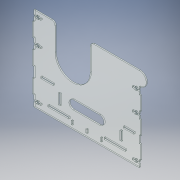
# Autodesk Inventor part: Lat_Izq_Caja
Saved by Autodesk Inventor 2019 (Build 230136000, 136)
## iProperties
Created: 2020-04-06
Part Number: Lat_Izq_Caja
Material: Generic
Document SubType Name: Modeling
Designer: Jurgen
Density: 1 g/cm^3
Appearance: Clear
Author: Jurgen
Autodesk Inventor part; units mm, degrees
ref_plane "YZ Plane" through (0, 0, 0) normal (1, 0, 0) x (0, 1, 0)
ref_plane "XZ Plane" through (0, 0, 0) normal (0, 1, 0) x (-1, 0, 0)
ref_plane "XY Plane" through (0, 0, 0) normal (0, 0, 1) x (1, 0, 0)
sketch "Sketch1" plane through (0, 0, 0) normal (0, 0, 1) x (1, 0, 0)
  line L0 (-150, -102.5) -> (40, -102.5) construction
  line L1 (-150, 5) -> (-150, -102.5) construction
  line L2 (-130, -37.5) -> (-95, -37.5)
  line L3 (-95, -37.5) -> (-95, -42.5)
  line L4 (-95, -42.5) -> (-130, -42.5)
  line L5 (-130, -37.5) -> (-130, -42.5)
  line L6 (-110, -97.5) -> (-50, -97.5)
  line L7 (-110, -97.5) -> (-110, -102.5)
  line L8 (-50, -102.5) -> (-110, -102.5)
  line L9 (-50, -97.5) -> (-50, -102.5)
  line L10 (110, -97.5) -> (50, -97.5)
  line L11 (110, -102.5) -> (50, -102.5)
  line L12 (50, -97.5) -> (50, -102.5)
  line L13 (110, -97.5) -> (110, -102.5)
  line L14 (95, -82.5) -> (95, -57.5)
  line L15 (95, -57.5) -> (100, -57.5)
  line L16 (100, -57.5) -> (100, -82.5)
  line L17 (95, -82.5) -> (100, -82.5)
  line L18 (-80, -82.5) -> (-80, -52.5)
  line L19 (-75, -52.5) -> (-75, -82.5)
  line L20 (-80, -52.5) -> (-75, -52.5)
  line L21 (-80, -82.5) -> (-75, -82.5)
  line L22 (135, -47.5) -> (105, -47.5)
  line L23 (135, -42.5) -> (105, -42.5)
  line L24 (105, -42.5) -> (105, -47.5)
  line L25 (135, -42.5) -> (135, -47.5)
  line L26 (-150, -97.5) -> (-150, -102.5) construction
  line L27 (-110, -102.5) -> (-150, -102.5) construction
  line L28 (150, -102.5) -> (110, -102.5) construction
  line L29 (150, -97.5) -> (150, -102.5) construction
  circle A0 centre (-39.5, 42.5) radius 33.5 construction
  circle A1 centre (-39.5, 42.5) radius 21 construction
  arc A2 (-27.2498, 9) -> (-19.0518, 13.2735) centre (-27.2498, 19) ccw construction
  line L30 (-27.2498, 9) -> (-81.7502, 9) construction
  line L31 (-1.6215, 38.2265) -> (-19.0518, 13.2735) construction
  arc A3 (6.5765, 42.5) -> (-1.6215, 38.2265) centre (6.5765, 32.5) ccw construction
  arc A4 (-89.9482, 13.2735) -> (-81.7502, 9) centre (-81.7502, 19) ccw construction
  line L32 (-89.9482, 13.2735) -> (-107.3785, 38.2265) construction
  arc A5 (-107.3785, 38.2265) -> (-115.5765, 42.5) centre (-115.5765, 32.5) ccw construction
  line L33 (-150, -102.5) -> (150, -102.5) construction
  line L34 (150, -102.5) -> (150, 117.5) construction
  line L35 (150, 117.5) -> (-150, 117.5) construction
  line L36 (-150, 117.5) -> (-150, -102.5) construction
  line L37 (-150, -102.5) -> (150, -102.5) construction
  line L38 (150, -102.5) -> (150, -122.5) construction
  line L39 (150, -122.5) -> (-150, -122.5)
  line L40 (-150, -122.5) -> (-150, -102.5) construction
  line L41 (-150, -122.5) -> (-150, 117.5)
  line L42 (150, 117.5) -> (150, -122.5)
  circle A6 centre (-39.5, 42.5) radius 50 construction
  line L43 (-150, 117.5) -> (-115.5765, 117.5) construction
  line L44 (-150, 117.5) -> (-120, 117.5)
  line L45 (46.1387, 117.5) -> (150, 117.5)
  line L46 (-89.5, 42.5) -> (10.5, 42.5) construction
  line L47 (-89.5, 42.5) -> (-89.5, 117.5) construction
  line L48 (10.5, 42.5) -> (10.5, 117.5) construction
  line L49 (-120, 117.5) -> (-89.5, 117.5)
  line L50 (-89.5, 117.5) -> (-89.5, 42.5)
  line L51 (46.1387, 117.5) -> (10.5, 117.5)
  line L52 (10.5, 117.5) -> (10.5, 42.5)
  arc A7 (-89.5, 42.5) -> (10.5, 42.5) centre (-39.5, 42.5) ccw
  point P0 (0, 0)
  point P1 (-84.8873, 21.524)
  point P2 (4.6333, 19)
  dimension "d2" = 300
  dimension "d3" = 220
  dimension "d4" = 300
  dimension "d5" = 20
  dimension "d6" = 100
  dimension "d7" = 30
  constraints: 106 end point, 14 point on circle, 8 centre point, 5 horizontal, 5 perpendicular, 5 point on line, 4 parallel, 2 collinear, 2 tangent, 1 coincident
  measures "d2" distance of L35.end L34.end
  measures "d3" distance of L34.end L33.end
  measures "d4" distance of L38.end L39.end
  measures "d5" distance of L37.end L38.end
  measures "d6" diameter of A6
  measures "d7" distance of L35.end L44.end
extrude "Extrusion1" add sketch "Sketch1" along normal blind 3.5
fillet "Fillet1" radius 10 2 edges at (-89.5, 117.5, 1.75) (10.5, 117.5, 1.75)
sketch "Sketch4" plane through (0, 0, 0) normal (0, 0, -1) x (-1, 0, 0)
  arc A0 (89.1717, 117.5) -> (79.1717, 107.5) centre (89.1717, 107.5) ccw construction
  line L0 (79.1717, 107.5) -> (79.1717, 42.6682) construction
  arc A1 (-0.8283, 42.6682) -> (79.1717, 42.6682) centre (39.1717, 42.6682) ccw construction
  line L1 (-0.8283, 42.6682) -> (-0.1119, 107.3893) construction
  arc A2 (-0.1119, 107.3893) -> (-10.1113, 117.5) centre (-10.1113, 107.5) ccw construction
  line L2 (-10.1113, 117.5) -> (-150, 117.5) construction
  line L3 (-150, 117.5) -> (-150, -122.5) construction
  line L4 (-150, -122.5) -> (150, -122.5) construction
  line L5 (150, -122.5) -> (150, 117.5) construction
  line L6 (150, 117.5) -> (89.1717, 117.5) construction
  line L7 (49.6717, -102.3318) -> (49.6717, -97.3318) construction
  line L8 (49.6717, -97.3318) -> (109.6717, -97.3318) construction
  line L9 (109.6717, -97.3318) -> (109.6717, -102.3318) construction
  line L10 (109.6717, -102.3318) -> (49.6717, -102.3318) construction
  line L11 (-110.3283, -97.3318) -> (-50.3283, -97.3318) construction
  line L12 (-50.3283, -97.3318) -> (-50.3283, -102.3318) construction
  line L13 (-50.3283, -102.3318) -> (-110.3283, -102.3318) construction
  line L14 (-110.3283, -102.3318) -> (-110.3283, -97.3318) construction
  line L15 (94.6717, -37.3318) -> (129.6717, -37.3318) construction
  line L16 (129.6717, -37.3318) -> (129.6717, -42.3318) construction
  line L17 (129.6717, -42.3318) -> (94.6717, -42.3318) construction
  line L18 (94.6717, -42.3318) -> (94.6717, -37.3318) construction
  line L19 (74.6717, -82.3318) -> (74.6717, -52.3318) construction
  line L20 (74.6717, -52.3318) -> (79.6717, -52.3318) construction
  line L21 (79.6717, -52.3318) -> (79.6717, -82.3318) construction
  line L22 (79.6717, -82.3318) -> (74.6717, -82.3318) construction
  line L23 (-135.3283, -42.3318) -> (-105.3283, -42.3318) construction
  line L24 (-105.3283, -42.3318) -> (-105.3283, -47.3318) construction
  line L25 (-105.3283, -47.3318) -> (-135.3283, -47.3318) construction
  line L26 (-135.3283, -47.3318) -> (-135.3283, -42.3318) construction
  line L27 (-95.3283, -82.3318) -> (-100.3283, -82.3318) construction
  line L28 (-100.3283, -82.3318) -> (-100.3283, -57.3318) construction
  line L29 (-100.3283, -57.3318) -> (-95.3283, -57.3318) construction
  line L30 (-95.3283, -57.3318) -> (-95.3283, -82.3318) construction
  line L31 (-150, 117.5) -> (-150, -122.5) construction
  arc A3 (-150, 77.5) -> (-160.9964, 80.7944) centre (-150, 97.5) ccw construction
  arc A4 (-150, 117.5) -> (-160.9964, 80.7944) centre (-150, 97.5) ccw
  line L32 (-150, 77.5) -> (-150, 62.5)
  line L33 (-150, 77.5) -> (-150, 117.5)
  line L34 (-150, -2.5) -> (-153.5, -2.5)
  line L35 (-153.5, -2.5) -> (-153.5, -42.5)
  line L36 (-153.5, -42.5) -> (-150, -42.5)
  line L37 (-150, -42.5) -> (-150, -2.5)
  line L38 (-150, -102.5) -> (-153.5, -102.5)
  line L39 (-153.5, -102.5) -> (-153.5, -62.5)
  line L40 (-153.5, -62.5) -> (-150, -62.5)
  line L41 (-150, -62.5) -> (-150, -102.5)
  line L42 (-150, 57.5) -> (-153.5, 57.5)
  line L43 (-153.5, 57.5) -> (-153.5, 17.5)
  line L44 (-153.5, 17.5) -> (-150, 17.5)
  line L45 (-150, 17.5) -> (-150, 57.5)
  line L46 (-150, -122.5) -> (-150, 117.5) construction
  line L47 (0, -122.5) -> (0, -42.5) construction
  line L48 (150, 87.5) -> (153.5, 87.5)
  line L49 (153.5, 87.5) -> (153.5, 47.5)
  line L50 (153.5, 47.5) -> (150, 47.5)
  line L51 (150, 47.5) -> (150, 87.5)
  line L52 (150, -122.5) -> (150, 117.5) construction
  line L53 (150, 17.5) -> (153.5, 17.5)
  line L54 (153.5, 17.5) -> (153.5, -22.5)
  line L55 (153.5, -22.5) -> (150, -22.5)
  line L56 (150, -22.5) -> (150, 17.5)
  line L57 (150, -52.5) -> (153.5, -52.5)
  line L58 (153.5, -52.5) -> (153.5, -92.5)
  line L59 (153.5, -92.5) -> (150, -92.5)
  line L60 (150, -92.5) -> (150, -52.5)
  arc A5 (-150, 117.5) -> (-150, 77.5) centre (-150, 97.5) ccw
  line L61 (-150, 117.5) -> (-150, -122.5) construction
  line L62 (-150, -122.5) -> (150, -122.5) construction
  point P0 (0, 0)
  dimension "d23" = 40
  dimension "d24" = 20
  dimension "d25" = 15
  dimension "d26" = 3.5
  dimension "d27" = 40
  dimension "d28" = 3.5
  dimension "d29" = 40
  dimension "d30" = 20
  dimension "d31" = 20
  dimension "d32" = 3.5
  dimension "d33" = 40
  dimension "d34" = 20
  dimension "d35" = 3.5
  dimension "d36" = 40
  dimension "d37" = 3.5
  dimension "d38" = 40
  dimension "d39" = 3.5
  dimension "d40" = 40
  dimension "d41" = 30
  dimension "d42" = 30
  dimension "d43" = 30
  constraints: 122 end point, 12 parallel, 12 point on circle, 8 point on line, 6 centre point, 6 horizontal, 6 perpendicular, 3 tangent, 1 midpoint, 1 vertical
  measures "d23" diameter of A3
  measures "d24" distance from line of L2 A3.centre
  measures "d25" distance of L32.start L32.end
  measures "d26" distance of L36.end L35.end
  measures "d27" distance of L35.end L34.end
  measures "d28" distance of L39.end L40.end
  measures "d29" distance of L38.end L39.end
  measures "d30" distance between parallel lines of L4 L38
  measures "d31" distance between parallel lines of L40 L36
  measures "d32" distance of L44.end L43.end
  measures "d33" distance of L43.end L42.end
  measures "d34" distance from line of L34.end L44
  measures "d35" distance of L49.end L50.end
  measures "d36" distance of L48.end L49.end
  measures "d37" distance of L54.end L55.end
  measures "d38" distance of L53.end L54.end
  measures "d39" distance of L58.end L59.end
  measures "d40" distance of L57.end L58.end
  measures "d41" distance between parallel lines of L4 L59
  measures "d42" distance between parallel lines of L57 L55
  measures "d43" distance between parallel lines of L53 L50
extrude "Extrusion3" add sketch "Sketch4" against normal blind 3.5
sketch "Sketch5" plane through (0, 0, 0) normal (0, 0, -1) x (-1, 0, 0)
  arc A0 (89.1717, 117.5) -> (79.1717, 107.5) centre (89.1717, 107.5) ccw construction
  line L0 (79.1717, 107.5) -> (79.1717, 42.6682) construction
  arc A1 (-0.8283, 42.6682) -> (79.1717, 42.6682) centre (39.1717, 42.6682) ccw construction
  line L1 (-0.8283, 42.6682) -> (-0.1119, 107.3893) construction
  arc A2 (-0.1119, 107.3893) -> (-10.1113, 117.5) centre (-10.1113, 107.5) ccw construction
  line L2 (-10.1113, 117.5) -> (-150, 117.5) construction
  arc A3 (-150, 117.5) -> (-150, 77.5) centre (-150, 97.5) ccw construction
  line L3 (-150, 77.5) -> (-150, 57.5) construction
  line L4 (-150, 57.5) -> (-153.5, 57.5) construction
  line L5 (-153.5, 57.5) -> (-153.5, 17.5) construction
  line L6 (-153.5, 17.5) -> (-150, 17.5) construction
  line L7 (-150, 17.5) -> (-150, -2.5) construction
  line L8 (-150, -2.5) -> (-153.5, -2.5) construction
  line L9 (-153.5, -2.5) -> (-153.5, -42.5) construction
  line L10 (-153.5, -42.5) -> (-150, -42.5) construction
  line L11 (-150, -42.5) -> (-150, -62.5) construction
  line L12 (-153.5, -62.5) -> (-150, -62.5) construction
  line L13 (-153.5, -102.5) -> (-153.5, -62.5) construction
  line L14 (-150, -102.5) -> (-153.5, -102.5) construction
  line L15 (-150, -102.5) -> (-150, -122.5) construction
  line L16 (-150, -122.5) -> (150, -122.5) construction
  line L17 (150, -122.5) -> (150, -92.5) construction
  line L18 (153.5, -92.5) -> (150, -92.5) construction
  line L19 (153.5, -52.5) -> (153.5, -92.5) construction
  line L20 (150, -52.5) -> (153.5, -52.5) construction
  line L21 (150, -52.5) -> (150, -22.5) construction
  line L22 (153.5, -22.5) -> (150, -22.5) construction
  line L23 (153.5, 17.5) -> (153.5, -22.5) construction
  line L24 (150, 17.5) -> (153.5, 17.5) construction
  line L25 (150, 17.5) -> (150, 47.5) construction
  line L26 (153.5, 47.5) -> (150, 47.5) construction
  line L27 (153.5, 87.5) -> (153.5, 47.5) construction
  line L28 (150, 87.5) -> (153.5, 87.5) construction
  line L29 (150, 87.5) -> (150, 117.5) construction
  line L30 (150, 117.5) -> (89.1717, 117.5) construction
  line L31 (49.6717, -102.3318) -> (49.6717, -97.3318) construction
  line L32 (49.6717, -97.3318) -> (109.6717, -97.3318) construction
  line L33 (109.6717, -97.3318) -> (109.6717, -102.3318) construction
  line L34 (109.6717, -102.3318) -> (49.6717, -102.3318) construction
  line L35 (-110.3283, -97.3318) -> (-50.3283, -97.3318) construction
  line L36 (-50.3283, -97.3318) -> (-50.3283, -102.3318) construction
  line L37 (-50.3283, -102.3318) -> (-110.3283, -102.3318) construction
  line L38 (-110.3283, -102.3318) -> (-110.3283, -97.3318) construction
  line L39 (94.6717, -37.3318) -> (129.6717, -37.3318) construction
  line L40 (129.6717, -37.3318) -> (129.6717, -42.3318) construction
  line L41 (129.6717, -42.3318) -> (94.6717, -42.3318) construction
  line L42 (94.6717, -42.3318) -> (94.6717, -37.3318) construction
  line L43 (74.6717, -82.3318) -> (74.6717, -52.3318) construction
  line L44 (74.6717, -52.3318) -> (79.6717, -52.3318) construction
  line L45 (79.6717, -52.3318) -> (79.6717, -82.3318) construction
  line L46 (79.6717, -82.3318) -> (74.6717, -82.3318) construction
  line L47 (-135.3283, -42.3318) -> (-105.3283, -42.3318) construction
  line L48 (-105.3283, -42.3318) -> (-105.3283, -47.3318) construction
  line L49 (-105.3283, -47.3318) -> (-135.3283, -47.3318) construction
  line L50 (-135.3283, -47.3318) -> (-135.3283, -42.3318) construction
  line L51 (-95.3283, -82.3318) -> (-100.3283, -82.3318) construction
  line L52 (-100.3283, -82.3318) -> (-100.3283, -57.3318) construction
  line L53 (-100.3283, -57.3318) -> (-95.3283, -57.3318) construction
  line L54 (-95.3283, -57.3318) -> (-95.3283, -82.3318) construction
  line L55 (-150, 77.5) -> (-150, 57.5) construction
  line L56 (-150, 65.5) -> (-130, 65.5) construction
  line L57 (-130, 65.5) -> (-130, 69.5) construction
  line L58 (-130, 69.5) -> (-150, 69.5) construction
  line L59 (-150, 69.5) -> (-150, 65.5) construction
  line L60 (-150, 67.5) -> (-130, 67.5) construction
  line L61 (-142, 63.5) -> (-138, 63.5) construction
  line L62 (-138, 63.5) -> (-138, 71.5) construction
  line L63 (-138, 71.5) -> (-142, 71.5) construction
  line L64 (-142, 71.5) -> (-142, 63.5) construction
  line L65 (-142, 63.5) -> (-138, 71.5) construction
  line L66 (-138, 63.5) -> (-142, 71.5) construction
  line L67 (-150, 69.5) -> (-150, 65.5)
  line L68 (-150, 65.5) -> (-142, 65.5)
  line L69 (-142, 65.5) -> (-142, 63.5)
  line L70 (-142, 63.5) -> (-138, 63.5)
  line L71 (-138, 63.5) -> (-138, 65.5)
  line L72 (-138, 65.5) -> (-130, 65.5)
  line L73 (-130, 65.5) -> (-130, 69.5)
  line L74 (-130, 69.5) -> (-138, 69.5)
  line L75 (-138, 69.5) -> (-138, 71.5)
  line L76 (-138, 71.5) -> (-142, 71.5)
  line L77 (-142, 71.5) -> (-142, 69.5)
  line L78 (-142, 69.5) -> (-150, 69.5)
  line L79 (-130, 9.5) -> (-150, 9.5) construction
  line L80 (-130, 9.5) -> (-138, 9.5)
  line L81 (-138, 11.5) -> (-142, 11.5) construction
  line L82 (-138, 11.5) -> (-142, 11.5)
  line L83 (-138, 9.5) -> (-138, 11.5)
  line L84 (-150, 7.5) -> (-130, 7.5) construction
  line L85 (-150, 5.5) -> (-130, 5.5) construction
  line L86 (-130, 5.5) -> (-130, 9.5) construction
  line L87 (-130, 5.5) -> (-130, 9.5)
  line L88 (-138, 5.5) -> (-130, 5.5)
  line L89 (-142, 3.5) -> (-138, 3.5) construction
  line L90 (-138, 3.5) -> (-142, 11.5) construction
  line L91 (-142, 3.5) -> (-138, 3.5)
  line L92 (-138, 3.5) -> (-138, 11.5) construction
  line L93 (-138, 3.5) -> (-138, 5.5)
  line L94 (-142, 3.5) -> (-138, 11.5) construction
  line L95 (-142, 5.5) -> (-142, 3.5)
  line L96 (-142, 11.5) -> (-142, 3.5) construction
  line L97 (-150, 5.5) -> (-142, 5.5)
  line L98 (-150, 9.5) -> (-150, 5.5) construction
  line L99 (-150, 9.5) -> (-150, 5.5)
  line L100 (-142, 9.5) -> (-150, 9.5)
  line L101 (-142, 11.5) -> (-142, 9.5)
  line L102 (-130, -108.5) -> (-150, -108.5) construction
  line L103 (-130, -108.5) -> (-138, -108.5)
  line L104 (-138, -106.5) -> (-142, -106.5) construction
  line L105 (-138, -106.5) -> (-142, -106.5)
  line L106 (-138, -108.5) -> (-138, -106.5)
  line L107 (-150, -110.5) -> (-130, -110.5) construction
  line L108 (-150, -112.5) -> (-130, -112.5) construction
  line L109 (-130, -112.5) -> (-130, -108.5) construction
  line L110 (-130, -112.5) -> (-130, -108.5)
  line L111 (-138, -112.5) -> (-130, -112.5)
  line L112 (-142, -114.5) -> (-138, -114.5) construction
  line L113 (-138, -114.5) -> (-142, -106.5) construction
  line L114 (-142, -114.5) -> (-138, -114.5)
  line L115 (-138, -114.5) -> (-138, -106.5) construction
  line L116 (-138, -114.5) -> (-138, -112.5)
  line L117 (-142, -114.5) -> (-138, -106.5) construction
  line L118 (-142, -112.5) -> (-142, -114.5)
  line L119 (-142, -106.5) -> (-142, -114.5) construction
  line L120 (-150, -112.5) -> (-142, -112.5)
  line L121 (-150, -108.5) -> (-150, -112.5) construction
  line L122 (-150, -108.5) -> (-150, -112.5)
  line L123 (-142, -108.5) -> (-150, -108.5)
  line L124 (-142, -106.5) -> (-142, -108.5)
  line L125 (150, 117.5) -> (89.1717, 117.5) construction
  line L126 (-150, -122.5) -> (150, -122.5) construction
  line L127 (150, -122.5) -> (150, 117.5) construction
  line L128 (150, 117.5) -> (-150, 117.5) construction
  line L129 (-150, 117.5) -> (-150, -122.5) construction
  line L130 (0, -122.5) -> (0, -40.5) construction
  line L131 (150, 17.5) -> (150, -2.5) construction
  line L132 (153.5, 17.5) -> (150, 17.5) construction
  line L133 (142, 98.5) -> (138, 98.5)
  line L134 (130, 100.5) -> (130, 104.5) construction
  line L135 (150, 100.5) -> (142, 100.5)
  line L136 (142, 104.5) -> (150, 104.5)
  line L137 (150, 104.5) -> (150, 100.5) construction
  line L138 (150, 104.5) -> (150, 100.5)
  line L139 (130, 100.5) -> (130, 104.5)
  line L140 (138, 100.5) -> (130, 100.5)
  line L141 (130, 104.5) -> (138, 104.5)
  line L142 (150, 100.5) -> (130, 100.5) construction
  line L143 (130, 104.5) -> (150, 104.5) construction
  line L144 (150, 102.5) -> (130, 102.5) construction
  line L145 (142, 98.5) -> (138, 98.5) construction
  line L146 (138, 98.5) -> (138, 100.5)
  line L147 (142, 100.5) -> (142, 98.5)
  line L148 (138, 104.5) -> (138, 106.5)
  line L149 (142, 106.5) -> (142, 104.5)
  line L150 (138, 106.5) -> (142, 106.5)
  line L151 (138, 106.5) -> (142, 106.5) construction
  line L152 (138, 98.5) -> (138, 106.5) construction
  line L153 (138, 98.5) -> (142, 106.5) construction
  line L154 (142, 98.5) -> (138, 106.5) construction
  line L155 (142, 106.5) -> (142, 98.5) construction
  line L156 (138, 30.5) -> (130, 30.5)
  line L157 (130, 34.5) -> (138, 34.5)
  line L158 (130, 30.5) -> (130, 34.5) construction
  line L159 (130, 30.5) -> (130, 34.5)
  line L160 (142, 30.5) -> (142, 28.5)
  line L161 (150, 30.5) -> (142, 30.5)
  line L162 (142, 28.5) -> (138, 28.5)
  line L163 (138, 28.5) -> (138, 30.5)
  line L164 (142, 28.5) -> (138, 28.5) construction
  line L165 (150, 34.5) -> (150, 30.5) construction
  line L166 (150, 34.5) -> (150, 30.5)
  line L167 (150, 32.5) -> (130, 32.5) construction
  line L168 (150, 30.5) -> (130, 30.5) construction
  line L169 (142, 34.5) -> (150, 34.5)
  line L170 (130, 34.5) -> (150, 34.5) construction
  line L171 (142, 36.5) -> (142, 34.5)
  line L172 (142, 36.5) -> (142, 28.5) construction
  line L173 (138, 28.5) -> (142, 36.5) construction
  line L174 (142, 28.5) -> (138, 36.5) construction
  line L175 (138, 28.5) -> (138, 36.5) construction
  line L176 (138, 34.5) -> (138, 36.5)
  line L177 (138, 36.5) -> (142, 36.5)
  line L178 (138, 36.5) -> (142, 36.5) construction
  line L179 (138, -109.5) -> (130, -109.5)
  line L180 (130, -105.5) -> (138, -105.5)
  line L181 (130, -109.5) -> (130, -105.5) construction
  line L182 (130, -109.5) -> (130, -105.5)
  line L183 (142, -109.5) -> (142, -111.5)
  line L184 (150, -109.5) -> (142, -109.5)
  line L185 (142, -111.5) -> (138, -111.5)
  line L186 (138, -111.5) -> (138, -109.5)
  line L187 (142, -111.5) -> (138, -111.5) construction
  line L188 (150, -105.5) -> (150, -109.5) construction
  line L189 (150, -105.5) -> (150, -109.5)
  line L190 (150, -107.5) -> (130, -107.5) construction
  line L191 (150, -109.5) -> (130, -109.5) construction
  line L192 (142, -105.5) -> (150, -105.5)
  line L193 (130, -105.5) -> (150, -105.5) construction
  line L194 (142, -103.5) -> (142, -105.5)
  line L195 (142, -103.5) -> (142, -111.5) construction
  line L196 (138, -111.5) -> (142, -103.5) construction
  line L197 (142, -111.5) -> (138, -103.5) construction
  line L198 (138, -111.5) -> (138, -103.5) construction
  line L199 (138, -105.5) -> (138, -103.5)
  line L200 (138, -103.5) -> (142, -103.5)
  line L201 (138, -103.5) -> (142, -103.5) construction
  line L202 (-150, -122.5) -> (150, -122.5) construction
  line L203 (150, -122.5) -> (150, -92.5) construction
  point P0 (0, 0)
  point P1 (-140, 67.5)
  point P2 (-140, 7.5)
  point P3 (-140, -110.5)
  point P4 (140, 102.5)
  point P5 (140, 32.5)
  point P6 (140, -107.5)
  dimension "d46" = 20
  dimension "d47" = 4
  dimension "d48" = 4
  dimension "d49" = 8
  dimension "d50" = 8
  dimension "d51" = 8
  dimension "d52" = 20
  dimension "d53" = 4
  dimension "d54" = 4
  dimension "d55" = 8
  dimension "d56" = 8
  dimension "d57" = 20
  dimension "d58" = 4
  dimension "d59" = 4
  dimension "d60" = 8
  dimension "d61" = 8
  dimension "d62" = 8
  dimension "d63" = 6
  dimension "d64" = 20
  dimension "d65" = 8
  dimension "d66" = 4
  dimension "d67" = 8
  dimension "d68" = 13
  dimension "d69" = 2
  dimension "d70" = 8
  dimension "d71" = 4
  dimension "d72" = 2
  dimension "d73" = 8
  dimension "d74" = 4
  dimension "d75" = 2
  dimension "d76" = 13
  dimension "d77" = 13
  dimension "d78" = 8
  dimension "d79" = 8
  constraints: 404 end point, 49 point on line, 25 midpoint, 23 perpendicular, 14 parallel, 8 point on circle, 7 horizontal, 4 centre point, 3 collinear, 3 vertical, 1 symmetric about line
  measures "d46" distance of L58.end L57.end
  measures "d47" distance of L57.end L56.end
  measures "d48" distance of L63.end L62.end
  measures "d49" distance of L62.end L61.end
  measures "d50" distance between parallel lines of L57 L62
  measures "d51" distance between parallel lines of L4 L68
  measures "d52" distance of L79.end L79.start
  measures "d53" distance of L79.start L85.end
  measures "d54" distance of L81.end L81.start
  measures "d55" distance of L81.start L89.end
  measures "d56" distance between parallel lines of L86 L92
  measures "d57" distance of L102.end L102.start
  measures "d58" distance of L102.start L108.end
  measures "d59" distance of L104.end L104.start
  measures "d60" distance of L104.start L112.end
  measures "d61" distance between parallel lines of L109 L115
  measures "d62" distance between parallel lines of L8 L85
  measures "d63" distance between parallel lines of L14 L123
  measures "d64" distance between parallel lines of L29 L134
  measures "d65" distance between parallel lines of L133 L151
  measures "d66" distance between parallel lines of L140 L141
  measures "d67" distance between parallel lines of L29 L155
  measures "d68" distance between parallel lines of L28 L135
  measures "d69" distance between parallel lines of L140 L133
  measures "d70" distance between parallel lines of L162 L178
  measures "d71" distance between parallel lines of L156 L157
  measures "d72" distance between parallel lines of L156 L162
  measures "d73" distance between parallel lines of L185 L201
  measures "d74" distance between parallel lines of L179 L180
  measures "d75" distance between parallel lines of L179 L185
  measures "d76" distance between parallel lines of L26 L169
  measures "d77" distance between parallel lines of L18 L193
  measures "d78" distance between parallel lines of L25 L172
  measures "d79" distance between parallel lines of L127 L183
extrude "Extrusion4" cut sketch "Sketch5" against normal blind 3.5
sketch "Sketch6" plane through (0, 0, 3.5) normal (0, 0, 1) x (1, 0, 0)
  line L0 (-150, -122.4999) -> (-150, -114.4999) construction
  line L1 (-150, -122.5) -> (150, -122.5) construction
  line L2 (-43.5, -112.5) -> (-43.5, -102.5)
  line L3 (-40, -102.5) -> (-40, -112.5)
  line L4 (-43.5, -102.5) -> (-40, -102.5)
  line L5 (-43.5, -112.5) -> (-40, -112.5)
  line L6 (-1.75, -112.5) -> (-1.75, -102.5)
  line L7 (-1.75, -102.5) -> (1.75, -102.5)
  line L8 (-1.75, -112.5) -> (1.75, -112.5)
  line L9 (1.75, -102.5) -> (1.75, -112.5)
  line L10 (40, -112.5) -> (40, -102.5)
  line L11 (40, -102.5) -> (43.5, -102.5)
  line L12 (40, -112.5) -> (43.5, -112.5)
  line L13 (43.5, -102.5) -> (43.5, -112.5)
  line L14 (-150, -109.5) -> (-150, -122.5) construction
  line L15 (-150, -122.5) -> (150, -122.5) construction
  line L16 (0, -122.5) -> (0, 0) construction
  line L17 (-50, -73.75) -> (50, -73.75)
  line L18 (50, -73.75) -> (50, -48.75)
  line L19 (50, -48.75) -> (-50, -48.75)
  line L20 (-50, -48.75) -> (-50, -73.75)
  line L21 (-50, -73.75) -> (50, -48.75) construction
  line L22 (50, -73.75) -> (-50, -48.75) construction
  point P0 (0, -61.25)
  dimension "d82" = 100
  dimension "d83" = 25
  constraints: 42 end point, 4 midpoint, 2 parallel, 1 horizontal, 1 perpendicular, 1 vertical
  measures "d82" distance of L19.end L18.end
  measures "d83" distance of L18.end L17.end
extrude "Extrusion5" cut sketch "Sketch6" against normal blind 3.5
fillet "Fillet2" radius 12.5 4 edges at (-50, -73.75, 1.75) (-50, -48.75, 1.75) (50, -48.75, 1.75) (50, -73.75, 1.75)
body "Solid1"
